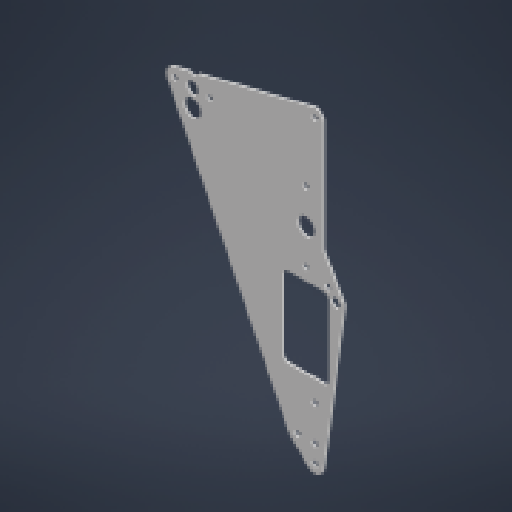
# Autodesk Inventor part: outer-tower-support-proto
Saved by Autodesk Inventor 2023.2 (Build 272271000, 271)
## iProperties
Created: 2023-03-21
Part Number: outer-tower-support-proto
Material: Generic
Document SubType Name: Modeling
Designer: Liam
Density: 1 g/cm^3
Appearance: Default
Author: Liam
Autodesk Inventor part; units mm, degrees
ref_plane "YZ Plane" through (0, 0, 0) normal (1, 0, 0) x (0, 1, 0)
ref_plane "XZ Plane" through (0, 0, 0) normal (0, 1, 0) x (-1, 0, 0)
ref_plane "XY Plane" through (0, 0, 0) normal (0, 0, 1) x (1, 0, 0)
sketch "Sketch1" plane through (0, 0, 0) normal (0, 0, 1) x (1, 0, 0)
  circle A0 centre (4.7625, -196.85) radius 2.1844 projected
  circle A1 centre (-84.1375, -17.4625) radius 2.1844 projected
  circle A2 centre (-58.7375, -17.4625) radius 2.1844 projected
  circle A3 centre (-71.4375, -30.1625) radius 1.4859 projected
  circle A4 centre (-71.4375, -30.1625) radius 6.35
  circle A5 centre (17.4625, -209.55) radius 2.1844 projected
  circle A6 centre (17.4625, -196.85) radius 2.1844 projected
  circle A7 centre (17.4625, 7.9375) radius 2.1844 projected
  line L0 (12.9724, -214.0401) -> (0.2724, -201.3401)
  line L1 (-0.9271, -199.6696) -> (-89.8271, -20.2821)
  line L2 (23.8125, 7.9375) -> (23.8125, -44.45)
  arc A8 (12.9724, -214.0401) -> (23.8125, -209.55) centre (17.4625, -209.55) ccw
  arc A9 (-0.9271, -199.6696) -> (0.2724, -201.3401) centre (4.7625, -196.85) ccw
  arc A10 (-85.6776, -11.3021) -> (-89.8271, -20.2821) centre (-84.1375, -17.4625) ccw
  arc A11 (23.8125, 7.9375) -> (15.9224, 14.0979) centre (17.4625, 7.9375) ccw
  line L3 (23.8125, -44.45) -> (23.8125, -71.9613)
  circle A12 centre (-71.4375, -17.4625) radius 2.1844
  line L4 (-85.6776, -11.3021) -> (-75.211, -8.6854)
  line L5 (15.9224, 14.0979) -> (-66.2619, -6.4482)
  arc A13 (-73.1895, -8.8477) -> (-67.9692, -7.5426) centre (-71.4375, -4.7625) ccw
  arc A14 (-66.2619, -6.4482) -> (-67.9692, -7.5426) centre (-65.4918, -9.5284) ccw
  arc A15 (-73.1895, -8.8477) -> (-75.211, -8.6854) centre (-74.4409, -11.7656) ccw
  circle A16 centre (-71.4375, -17.4625) radius 4.445
  circle A17 centre (17.4625, -171.45) radius 2.1844 projected
  circle A18 centre (11.1125, -88.9) radius 2.2098
  circle A19 centre (11.1125, -63.5) radius 2.1844 projected
  circle A20 centre (11.1125, -38.1) radius 2.1844 projected
  line L6 (34.586, -103.8945) -> (30.8299, -104.047) projected
  line L7 (36.332, -100.5653) -> (34.586, -103.8945) projected
  line L8 (30.8299, -104.047) -> (28.8198, -100.8704) projected
  line L9 (28.8198, -100.8704) -> (30.5657, -97.5412) projected
  line L10 (30.5657, -97.5412) -> (34.3218, -97.3887) projected
  line L11 (34.3218, -97.3887) -> (36.332, -100.5653) projected
  line L12 (34.586, -103.8945) -> (30.5657, -97.5412)
  circle A21 centre (26.9875, -93.6245) radius 2.2098
  circle A22 centre (11.1125, -63.5) radius 6.35
  line L13 (38.0767, -97.5456) -> (24.2371, -73.5474)
  arc A23 (27.6125, -101.95) -> (24.0125, -98.35) centre (24.0125, -101.95) ccw projected
  arc A24 (-1.7875, -98.35) -> (-5.3875, -101.95) centre (-1.7875, -101.95) ccw projected
  arc A25 (-5.3875, -152.05) -> (-1.7875, -155.65) centre (-1.7875, -152.05) ccw projected
  arc A26 (24.0125, -155.65) -> (27.6125, -152.05) centre (24.0125, -152.05) ccw projected
  line L14 (-5.8515, -152.05) -> (-5.8515, -101.95)
  line L15 (-1.7875, -97.886) -> (24.0125, -97.886)
  line L16 (24.0125, -156.114) -> (-1.7875, -156.114)
  line L17 (28.0765, -152.05) -> (28.0765, -101.95)
  arc A27 (24.0125, -156.114) -> (28.0765, -152.05) centre (24.0125, -152.05) ccw
  arc A28 (-5.8515, -152.05) -> (-1.7875, -156.114) centre (-1.7875, -152.05) ccw
  arc A29 (-1.7875, -97.886) -> (-5.8515, -101.95) centre (-1.7875, -101.95) ccw
  arc A30 (28.0765, -101.95) -> (24.0125, -97.886) centre (24.0125, -101.95) ccw
  line L18 (23.8125, -209.55) -> (38.865, -101.5948)
  arc A31 (38.865, -101.5948) -> (38.0767, -97.5456) centre (32.5759, -100.7179) ccw
  arc A32 (23.8125, -71.9613) -> (24.2371, -73.5474) centre (26.9875, -71.9613) ccw
  point P0 (0, 0)
  point P1 (-74.0123, -8.3858)
  point P2 (-67.4605, -6.7478)
  point P3 (16.6133, -60.3277)
  dimension "d39" = 12.7
  dimension "d13" = 12.7
  dimension "d30" = 4.3688
  dimension "d32" = 3.175
  dimension "d33" = 8.89
  dimension "d34" = 4.4196
  dimension "d38" = 4.4196
  dimension "d44" = 3.175
  constraints: 28 point on circle, 26 end point, 18 centre point, 11 tangent, 7 coincident, 4 point on line, 1 equal radius, 1 vertical, 8 other
  measures "d13" diameter of A4
  measures "d30" diameter of A12
  measures "d32" radius of A14
  measures "d33" diameter of A16
  measures "d34" diameter of A18
  measures "d38" diameter of A21
  measures "d44" radius of A32
extrude "Extrusion5" add sketch "Sketch1" along normal blind 1.524 contours L0 A9 L1 A10 L4 A15 A13 A14 L5 A11 L2 L3 A32 L13 A31 L18 A8
body "Solid5"
